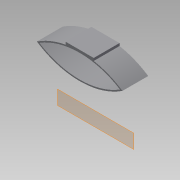
# Autodesk Inventor part: 07_Feder
Saved by Autodesk Inventor 2015 (Build 190159000, 159)
## iProperties
Created: 2015-12-20
Part Number: 07_Feder
Material: Generisch
Document SubType Name: Modeling
Designer: Bene
Density: 1 g/cm^3
Appearance: Vorgabe
Author: Bene
Autodesk Inventor part; units mm, degrees
ref_plane "YZ Plane" through (0, 0, 0) normal (1, 0, 0) x (0, 1, 0)
ref_plane "XZ Plane" through (0, 0, 0) normal (0, 1, 0) x (-1, 0, 0)
ref_plane "XY Plane" through (0, 0, 0) normal (0, 0, 1) x (1, 0, 0)
ref_plane "Arbeitsebene1" through (-23.7843, -50.4597, 67.3862) normal (0, -1, 0) x (-1, 0, 0)
sketch "Skizze1" plane through (-23.7843, -50.4597, 67.3862) normal (0, -1, 0) x (-1, 0, 0)
  arc A0 (-13.7675, -44.4592) -> (52.565, -44.4592) centre (19.3987, 5.5408) ccw
  arc A1 (52.565, -44.4592) -> (-13.7675, -44.4592) centre (19.3987, -94.4592) ccw
  arc A2 (-12.8526, -43.8642) -> (51.65, -43.8642) centre (19.3987, 5.5408) ccw
  arc A3 (51.65, -45.0542) -> (-12.8526, -45.0542) centre (19.3987, -94.4592) ccw
  line L0 (30.3074, -55.4592) -> (8.49, -55.4592)
  line L1 (8.49, -55.4592) -> (8.49, -53.4592)
  line L2 (8.49, -53.4592) -> (30.3074, -53.4592)
  line L3 (30.3074, -53.4592) -> (30.3074, -55.4592)
  line L4 (30.3074, -55.4592) -> (8.49, -53.4592) construction
  line L5 (8.49, -55.4592) -> (30.3074, -53.4592) construction
  point P0 (-23.7843, 67.3862)
  point P1 (50.7196, -44.4592)
  point P2 (-11.9222, -44.4592)
  point P3 (19.3987, -54.4592)
  dimension "d0" = 120
  dimension "d1" = 120
  dimension "d2" = 100
  dimension "d3" = 0
  dimension "d4" = 1
  dimension "d5" = 1
  constraints: 18 point on circle, 12 end point, 4 centre point, 2 midpoint, 2 parallel, 1 horizontal, 1 perpendicular
  measures "d0" diameter of A0
  measures "d1" diameter of A1
  measures "d2" distance of A0.centre A1.centre
  measures "d3" horizontal distance of A0.centre A1.centre
  measures "d4" radial gap between concentric circles of A0 A2
  measures "d5" radial gap between concentric circles of A1 A3
extrude "Extrusion1" add sketch "Skizze1" along normal blind 20 contours A1 A2 A3 A0 | A3 A2 L2 A0 | A1 A2 A3 | L2 A0 | A0 L3 L0 L1 | A1 A0 A3 A2 | L2 A2 A3 A0
